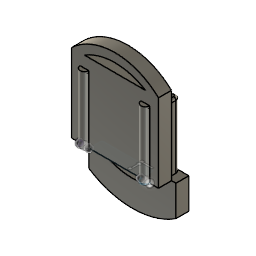
quick_swap_sliding_lock (Autodesk Fusion 360 design; units mm, degrees)
Autodesk Fusion 360 part; units mm, degrees
sketch "Sketch1" plane through (0, 0, 0) normal (1, 0, 0) x (0, 1, 0)
sketch "Sketch2" plane through (0, 0, 0) normal (0, 1, 0) x (1, 0, 0)
  line L0 (0, 0) -> (0, -90)
  line L1 (100, 0) -> (100, -90)
  arc A0 (0, -90) -> (100, -90) centre (50, -37.5) ccw
  line L2 (0, 0) -> (10, 0)
  line L3 (10, 0) -> (10, -75)
  line L4 (10, -75) -> (15, -75)
  line L5 (15, -75) -> (15, 0)
  line L6 (15, 0) -> (10, 0)
  line L7 (100, 0) -> (90, 0)
  line L8 (90, 0) -> (90, -75)
  line L9 (90, -75) -> (85, -75)
  line L10 (85, -75) -> (85, 0)
  line L11 (85, 0) -> (90, 0)
  line L12 (10, -75) -> (0, -75)
  line L13 (90, -75) -> (100, -75)
  line L14 (0, -90) -> (100, -90)
  arc A1 (15, -90) -> (85, -90) centre (50, -33.75) ccw
  line L15 (15, -75) -> (15, -90)
  line L16 (85, -75) -> (85, -90)
  line L17 (15, -75) -> (20, -75)
  line L18 (20, -75) -> (20, 0)
  line L19 (20, 0) -> (15, 0)
  line L20 (85, -75) -> (80, -75)
  line L21 (80, -75) -> (80, 0)
  line L22 (80, 0) -> (85, 0)
  line L23 (20, -75) -> (80, -75)
  line L24 (80, 0) -> (20, 0)
  dimension "d1" = 90
  dimension "d2" = 10
  dimension "d3" = 10
  constraint coincident L0.start L2.start
  constraint vertical L0
  constraint perpendicular L0 L2
  constraint perpendicular L2 L3
  constraint perpendicular L3 L4
  constraint perpendicular L4 L5
  constraint perpendicular L3 L6
  constraint perpendicular L1 L7
  constraint perpendicular L4 L8
  constraint perpendicular L8 L9
  constraint perpendicular L9 L10
  constraint perpendicular L10 L11
  constraint coincident L0 L12.end
  constraint perpendicular L0 L12
  constraint coincident L1 L13.end
  constraint perpendicular L1 L13
  constraint perpendicular L1 L14
  constraint coincident L14 A1.end
  constraint coincident L14 A1.start
  constraint perpendicular L14 L15
  constraint perpendicular L14 L16
  constraint perpendicular L5 L17
  constraint perpendicular L4 L18
  constraint perpendicular L5 L19
  constraint perpendicular L10 L20
  constraint perpendicular L20 L21
  constraint perpendicular L21 L22
  constraint perpendicular L21 L23
  constraint perpendicular L18 L24
  measures "d1" distance of L0.start L0.end
  measures "d2" distance of L0.start L2.end
  measures "d3" distance of L1.start L7.end
extrude "Extrude1" add sketch "Sketch2" along normal blind 15 contours L0 L2 L3 L12 | L0 L4 L12 L14 L15 | A0 L14 A1 | L1 L9 L13 L14 L16 | L14 L15 L16 L17 L20 L23 | L18 L21 L23 L24 | L1 L7 L8 L13 makes body 1
sketch "Sketch3" plane through (0, 0, 0) normal (0, 1, 0) x (1, 0, 0)
mirror "Mirror1" about plane through (0, 0, 0) normal (0, 1, 0) of bodies 1 makes body 2
move_body "Move1" bodies 2 to x (1, 0, 0) y (0, 1, 0) z (0, 0, 1) at (0, -75, 0)
move_body "Move2" bodies 2 to x (-1, 0, 0) y (0, 1, 0) z (0, 0, -1) at (110, 0, 110)
scale "Scale1" factor 1 about (90, -75, 35) bodies 2
sketch "Sketch4" plane through (0, -90, 0) normal (0, -1, 0) x (1, 0, 0)
  arc A0 (25, 20) -> (95, 20) centre (60, 76.25) ccw
  line L0 (25, 20) -> (95, 20)
  line L1 (20, 110) -> (10, 110)
  line L2 (10, 110) -> (10, 20)
  arc A1 (10, 20) -> (110, 20) centre (60, 72.5) ccw
  line L3 (110, 20) -> (110, 110)
  line L4 (110, 110) -> (100, 110)
  line L5 (100, 110) -> (100, 35)
  line L6 (100, 35) -> (90, 35)
  line L7 (90, 35) -> (90, 110)
  line L8 (90, 110) -> (30, 110)
  line L9 (30, 110) -> (30, 35)
  line L10 (30, 35) -> (20, 35)
  line L11 (20, 35) -> (20, 110)
  line L12 (30, 35) -> (90, 35)
  line L13 (90, 110) -> (30, 110)
  constraint coincident L9.end L10.start
  constraint coincident L6.end L7.start
  constraint coincident L7.end L8.start
  constraint coincident L8.end L9.start
extrude "Extrude2" cut sketch "Sketch4" against normal blind 30 contours L7 L8 L9 L12 L13 bodies 2
move_body "Move3" bodies 2 to x (1, 0, 0) y (0, 1, 0) z (0, 0, 1) at (-10, 110, -35)
sketch "Sketch5" plane through (0, 35, 0) normal (0, 1, 0) x (-1, 0, 0)
  line L0 (-10, 0) -> (-90, 0)
  line L1 (-90, 0) -> (-90, 75)
  line L2 (-90, 75) -> (-100, 75)
  line L3 (-100, 75) -> (-100, -15)
  arc A0 (-100, -15) -> (0, -15) centre (-50, 37.5) ccw
  line L4 (0, -15) -> (0, 75)
  line L5 (0, 75) -> (-10, 75)
  line L6 (-10, 75) -> (-10, 0)
  arc A1 (-85, -15) -> (-15, -15) centre (-50, 41.25) ccw
  line L7 (-85, -15) -> (-15, -15)
  line L8 (-10, 75) -> (-10, 0)
  line L9 (-20, 75, -20) -> (-20, 0, -20)
  line L10 (-90, 75) -> (-90, 0)
  line L11 (-90, 0) -> (-80, 0)
  line L12 (-80, 0) -> (-80, 75)
  line L13 (-80, 75) -> (-90, 75)
  line L14 (-10, 0) -> (-20, 0)
  line L15 (-10, 75) -> (-20, 75)
  line L16 (-20, 75) -> (-20, 0)
  point P0 (-20, 75)
  point P1 (-20, 0)
  dimension "d11" = 75
  dimension "d12" = 10
  dimension "d13" = 75
  dimension "d14" = 10
  dimension "d15" = 10
  constraint vertical L8
  constraint coincident L5.end L6.start
  constraint coincident P0 L15.end
  constraint coincident P1 L14.end
  constraint coincident L1.end L2.start
  constraint coincident L0.end L1.start
  constraint perpendicular L3 L11
  constraint perpendicular L11 L12
  constraint perpendicular L8 L14
  constraint perpendicular L6 L15
  measures "d11" distance of L5.end L0.start
  measures "d12" distance of L0.end L11.end
  measures "d13" distance of L11.end L12.end
  measures "d14" distance of L0.start P1
  measures "d15" distance of L5.end P0
sketch "Sketch6" plane through (0, 35, 0) normal (0, 1, 0) x (-1, 0, 0)
  line L0 (-10, 0) -> (0, 0)
  line L1 (0, 0) -> (0, 75)
  line L2 (0, 75) -> (-10, 75)
  line L3 (-10, 75) -> (-10, 0)
  line L4 (-100, 75) -> (-100, -15)
  line L5 (-90, 0) -> (-100, 0)
  line L6 (-100, 75) -> (-90, 75)
  line L7 (-90, 75) -> (-90, 0)
  line L8 (-100, 0) -> (-100, 75)
  point P0 (-10, 0)
  point P1 (0, 75)
  point P2 (-10, 75)
  point P3 (-10, 0)
  point P4 (-90, 0)
  point P5 (-90, 75)
  constraint coincident P3 P0
  constraint coincident L0.end L1.start
  constraint coincident P1 L1.end
  constraint coincident P2 L2.end
  constraint coincident P4 L5.start
  constraint coincident L4 L5.end
  constraint perpendicular L3 L5
  constraint coincident L4.start L6.start
  constraint coincident P5 L6.end
extrude "Extrude3" cut sketch "Sketch6" against normal blind 15 bodies 2
extrude "Extrude4" add sketch "Sketch5" against normal blind 15 contours L0 L6 L8 L14 L15 L16 | L0 L1 L10 L11 L12 L13 bodies 2
fillet "Fillet1" radius 5 6 edges at (80, 20, 37.5) (90, 20, 37.5) (85, 20, 75) (15, 20, 75) (20, 20, 37.5) (10, 20, 37.5) on bodies 2
fillet "Fillet2" radius 2.5 6 edges at (80, 15, 37.5) (85, 15, 75) (90, 15, 37.5) (20, 15, 37.5) (10, 15, 37.5) (15, 15, 75) on bodies 1
fillet "Fillet3" radius 2.5 8 edges at (20, 30, 75) (15, 20, 75) (10, 30, 75) (90, 30, 75) (85, 20, 75) (80, 30, 75) (85, 35, 75) (15, 35, 75) on bodies 2
move_face "OffsetFaces1" offset -5 2 faces at (96.6667, 26.6667, 0) (3.3333, 26.6667, 0) on bodies 2
move_face "OffsetFaces2" offset -5 2 faces at (14.1667, 27.5, 75) (84.1667, 27.5, 75) on bodies 2
move_face "OffsetFaces3" offset -5 1 faces at (40, 28.3333, 0) on bodies 2
fillet "Fillet4" radius 5 8 edges at (80, 35, 31.25) (80.7322, 34.2678, 69.2678) (89.2678, 34.2678, 69.2678) (90, 35, 31.25) (10.7322, 34.2678, 69.2678) (10, 35, 31.25) (19.2678, 34.2678, 69.2678) (20, 35, 31.25) on bodies 2
sketch "Sketch7" plane through (0, 0, 0) normal (0, 0, -1) x (1, 0, 0)
  arc A0 (20, -12.5) -> (22.5, -15) centre (22.5, -12.5) ccw
  line L0 (22.5, -15) -> (77.5, -15)
  arc A1 (77.5, -15) -> (80, -12.5) centre (77.5, -12.5) ccw
  line L1 (80, -12.5) -> (80, 0)
  line L2 (80, 0) -> (20, 0)
  line L3 (20, 0) -> (20, -12.5)
  arc A2 (20, 0) -> (10, 0) centre (15, 0) ccw
  arc A3 (89.9707, 0) -> (80, 0) centre (84.9854, 0) ccw
  point P0 (10, 0)
  constraint tangent L3 A2
  constraint coincident L2.end L3.start
  constraint coincident P0 A2.end
  constraint tangent L1 A3
  constraint coincident L1.end L2.start
sketch "Sketch8" plane through (0, 0, 0) normal (0, 0, 1) x (1, 0, 0)
  arc A0 (80, 0) -> (89.9707, 0) centre (84.9854, 0) ccw
  line L0 (90, 0) -> (80, 0)
  line L1 (10, 0) -> (20, 0)
  arc A1 (10, 0) -> (20, 0) centre (15, 0.0147) ccw
  point P0 (90, 0)
  point P1 (10, 0)
  point P2 (20, 0)
  constraint coincident P0 L0.start
  constraint coincident A0 L0.end
  constraint coincident P1 L1.start
  constraint coincident P2 L1.end
extrude "Extrude5" add sketch "Sketch8" along normal blind 77 separate body makes body 3 at (12.9472, -4.5445, 51.3333) makes body 4 at (85.1097, -4.9838, 51.3333)
sketch "Sketch9" plane through (0, 0, 0) normal (0, 0, -1) x (1, 0, 0)
  arc A0 (89.9707, 0) -> (80, 0) centre (84.9854, 0) ccw
  line L0 (80, 0) -> (89.9707, 0)
  line L1 (89.9707, 0) -> (80, 0)
  line L2 (89.9707, 0) -> (80, 0)
  arc A1 (89.9707, 0) -> (80, 0) centre (84.9854, -1.8857) ccw
  line L3 (20, 0) -> (10, 0)
  arc A2 (20, 0) -> (10, 0) centre (15, -1.9069) ccw
  point P0 (20, 0)
  point P1 (10, 0)
  constraint coincident A0.start L0.end
  constraint coincident A0.end L0.start
  constraint coincident P0 L3.start
  constraint coincident P1 L3.end
extrude "Extrude6" cut sketch "Sketch9" against normal blind 75 contours L0 L1 L2 A1 | L3 A2 bodies 3 4
move_face "OffsetFaces4" offset 20 1 faces at (2.4737, 25, -17.2495) on bodies 2
named bodies: "end_arm", "gripper"
